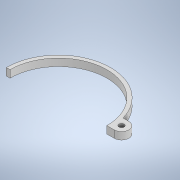
# Autodesk Inventor part: claw
Saved by Autodesk Inventor 2020 (Build 240168000, 168)
## iProperties
Created: 2020-03-11
Part Number: claw
Material: Generic
Document SubType Name: Modeling
Designer: cs1874
Density: 1 g/cm^3
Appearance: Default
Author: cs1874
Autodesk Inventor part; units mm, degrees
ref_plane "YZ Plane" through (0, 0, 0) normal (1, 0, 0) x (0, 1, 0)
ref_plane "XZ Plane" through (0, 0, 0) normal (0, 1, 0) x (-1, 0, 0)
ref_plane "XY Plane" through (0, 0, 0) normal (0, 0, 1) x (1, 0, 0)
sketch "Sketch1" plane through (0, 0, 0) normal (0, 1, 0) x (-1, 0, 0)
  circle A0 centre (0, 0) radius 1.75
  circle A1 centre (0, 0) radius 5
  line L0 (0, 5) -> (10, 5)
  line L1 (10, 5) -> (10, -5)
  line L2 (10, -5) -> (0, -5)
  line L3 (0, -5) -> (0, 5)
  line L4 (10, 5) -> (38, 5)
  line L5 (10, -5) -> (38, -5)
  circle A2 centre (38, 5) radius 33
  arc A3 (2.5, 5) -> (73.5, 5) centre (38, 5) ccw
  line L6 (38, 5) -> (73.5, 5)
  point P0 (3.9376, -5)
  point P1 (71, 5)
  point P2 (5, 5)
  dimension "d1" = 10
  dimension "d0" = 3.5
  dimension "d2" = 10
  dimension "d3" = 28
  dimension "d4" = 28
  dimension "d5" = 66
  dimension "d6" = 71
  constraints: 14 end point, 4 coincident, 4 horizontal, 3 centre point, 2 parallel, 2 point on circle, 1 perpendicular, 1 point on line, 3 other
  measures "d0" diameter of A0
  measures "d2" distance of L1.end L2.end
  measures "d3" distance of L0.end L4.end
  measures "d4" distance of L1.end L5.end
  measures "d5" diameter of A2
  measures "d6" diameter of A3
extrude "Extrusion1" add sketch "Sketch1" along normal blind 5 contours A0 L3 A1 A3 | A0 L3 A1 | L0 A3 A1 | A1 A3 L2 | A3 L0 A2 L2 A1 | A1 A3 | L2 A2 L6 A3
body "Solid1"
